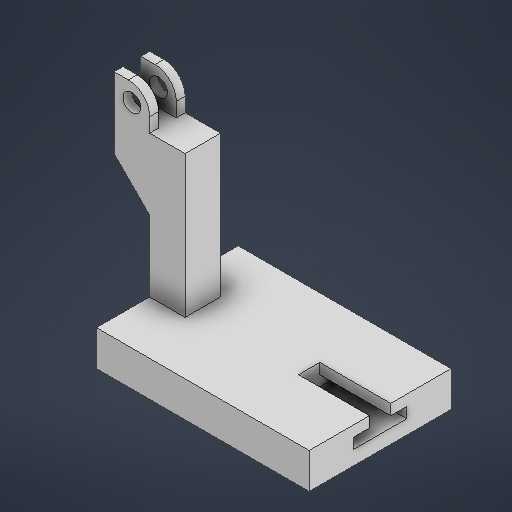
# Autodesk Inventor part: Press_Base
Saved by Autodesk Inventor 2026.1 (Build 301233020, 233B)
## iProperties
Created: 2025-09-29
Part Number: Press_Base
Material: Generic
Document SubType Name: Modeling
Designer: Gamec
Density: 1 g/cm^3
Appearance: Default
Author: Gamec
Autodesk Inventor part; units mm, degrees
ref_plane "YZ Plane" through (0, 0, 0) normal (1, 0, 0) x (0, 1, 0)
ref_plane "XZ Plane" through (0, 0, 0) normal (0, 1, 0) x (-1, 0, 0)
ref_plane "XY Plane" through (0, 0, 0) normal (0, 0, 1) x (1, 0, 0)
sketch "Sketch1" plane through (0, 0, 0) normal (0, 1, 0) x (-1, 0, 0)
  line L0 (-38.1, 25.4) -> (38.1, 25.4)
  line L1 (38.1, 25.4) -> (38.1, -25.4)
  line L2 (38.1, -25.4) -> (-38.1, -25.4)
  line L3 (-38.1, -25.4) -> (-38.1, 25.4)
  line L4 (-38.1, 25.4) -> (38.1, -25.4) construction
  line L5 (38.1, 25.4) -> (-38.1, -25.4) construction
  point P0 (0, 0)
  dimension "d0" = 76.2
  dimension "d1" = 50.8
  constraints: 12 end point, 2 midpoint, 2 parallel, 1 horizontal, 1 perpendicular
  measures "d0" distance of L1.end L2.end
  measures "d1" distance of L0.end L1.end
extrude "Extrusion1" add sketch "Sketch1" along normal blind 12.7
sketch "Sketch2" plane through (0, 12.7, 0) normal (0, 1, 0) x (1, 0, 0)
  line L0 (-38.1, 25.4) -> (-38.1, -25.4) projected
  line L1 (-38.1, 6.35) -> (-25.4, 6.35)
  line L2 (-25.4, 6.35) -> (-25.4, -6.35)
  line L3 (-25.4, -6.35) -> (-38.1, -6.35)
  line L4 (-38.1, -6.35) -> (-38.1, 6.35)
  point P0 (0, 0)
  dimension "d4" = 12.7
  dimension "d5" = 12.7
  dimension "d6" = 6.35
  constraints: 8 end point, 2 parallel, 1 horizontal, 1 perpendicular, 1 point on line
  measures "d4" distance of L2.end L3.end
  measures "d5" distance of L1.end L2.end
  measures "d6" distance from line of point (0, 0) L3
extrude "Extrusion2" add sketch "Sketch2" along normal blind 50.8
sketch "Sketch4" plane through (-38.1, 12.7, 6.35) normal (0, 0, 1) x (1, 0, 0)
  line L0 (0, 0) -> (0, 50.8) projected
  line L1 (0, 38.1) -> (-12.7, 38.1)
  line L2 (-12.7, 38.1) -> (-12.7, 63.5)
  line L3 (-12.7, 63.5) -> (0, 63.5)
  line L4 (0, 63.5) -> (0, 38.1)
  line L5 (0, 50.8) -> (12.7, 50.8) projected
  line L6 (-12.7, 38.1) -> (0, 25.4)
  circle A0 centre (-6.35, 57.15) radius 3.175
  point P0 (38.1, -12.7)
  dimension "d13" = 12.7
  dimension "d14" = 25.4
  dimension "d15" = 12.7
  dimension "d22" = 6.35
  dimension "d23" = 6.35
  dimension "d24" = 6.35
  constraints: 10 end point, 2 parallel, 1 centre point, 1 horizontal, 1 midpoint, 1 perpendicular, 1 point on line
  measures "d13" distance of L2.end L3.end
  measures "d14" distance of L1.end L2.end
  measures "d15" distance between parallel lines of L5 L1
  measures "d22" diameter of A0
  measures "d23" distance from line of L3 A0.centre
  measures "d24" distance from line of L4 A0.centre
extrude "Extrusion4" add sketch "Sketch4" against normal blind 12.7
sketch "Sketch5" plane through (-50.8, 76.2, 6.35) normal (0, 1, 0) x (1, 0, 0)
  line L0 (0, 0) -> (0, 12.7) projected
  line L1 (12.7, 12.7) -> (12.7, 0) projected
  line L2 (0, 9.525) -> (12.7, 9.525)
  line L3 (12.7, 9.525) -> (12.7, 3.175)
  line L4 (12.7, 3.175) -> (0, 3.175)
  line L5 (0, 3.175) -> (0, 9.525)
  line L6 (12.7, 0) -> (0, 0) projected
  point P0 (50.8, 6.35)
  point P1 (0, 3.175)
  dimension "d18" = 6.35
  dimension "d19" = 3.175
  constraints: 8 end point, 2 parallel, 2 point on line, 1 horizontal, 1 perpendicular
  measures "d18" distance of L2.end L3.end
  measures "d19" distance between parallel lines of L6 L4
extrude "Extrusion5" cut sketch "Sketch5" against normal blind 12.7 contours L0 L2 L1 L4
sketch "Sketch6" plane through (38.1, 0, 25.4) normal (1, 0, 0) x (0, 0, -1)
  line L0 (15.875, 8.89) -> (34.925, 8.89)
  line L1 (34.925, 8.89) -> (34.925, 5.08)
  line L2 (34.925, 5.08) -> (15.875, 5.08)
  line L3 (15.875, 5.08) -> (15.875, 8.89)
  line L4 (50.8, 0) -> (50.8, 12.7) projected
  line L5 (0, 12.7) -> (50.8, 12.7) projected
  line L6 (21.59, 8.89) -> (29.21, 8.89)
  line L7 (29.21, 8.89) -> (29.21, 12.7)
  line L8 (29.21, 12.7) -> (21.59, 12.7)
  line L9 (21.59, 12.7) -> (21.59, 8.89)
  point P0 (25.4, 0)
  point P1 (29.21, 12.7)
  dimension "d25" = 19.05
  dimension "d26" = 3.81
  dimension "d27" = 15.875
  dimension "d28" = 3.81
  dimension "d29" = 7.62
  dimension "d30" = 3.81
  dimension "d31" = 5.715
  constraints: 16 end point, 4 parallel, 2 horizontal, 2 perpendicular, 1 point on line
  measures "d25" distance of L1.end L2.end
  measures "d26" distance of L0.end L1.end
  measures "d27" distance between parallel lines of L4 L1
  measures "d28" distance between parallel lines of L5 L0
  measures "d29" distance of L8.end L7.end
  measures "d30" distance of L7.end L6.end
  measures "d31" distance between parallel lines of L1 L7
extrude "Extrusion6" cut sketch "Sketch6" against normal blind 25.4
fillet "Fillet1" radius 7.62 2 edges at (-38.1, 76.2, 4.7625) (-38.1, 76.2, -4.7625)
body "Solid1"
